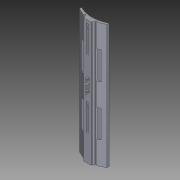
# Autodesk Inventor part: 3213_Bed Holder
Saved by Autodesk Inventor 2020 (Build 240168000, 168)
## iProperties
Created: 2019-06-26
Part Number: 3213_Bed Holder
Material: Acetal Resin, White
Document SubType Name: Sheet Metal
Designer: MPI
Density: 1.425 g/cm^3
Sheet Metal Rule: Default_mm
Appearance: Smooth - White
Mass: 236.302 g
Surface Area: 644.505 cm^2
Volume: 165.826 cm^3
Author: MPI
Autodesk Inventor part; units mm, degrees
sketch "Sketch1" plane through (0, 0, 0) normal (0, 0, 1) x (1, 0, 0)
  line L0 (0, 0) -> (-20.6965, 9.6509) construction
  line L1 (0, 0) -> (0, -60.6509) construction
  line L2 (0, 0) -> (-23.2307, -49.8183) construction
  line L3 (0, 0) -> (21.0241, 9.8037) construction
  line L4 (0, 0) -> (21.5225, -46.1553) construction
  line L5 (0, 0) -> (0, 48) construction
  arc A0 (-36, -19.5) -> (36, -19.5) centre (0, 48) ccw
  line L6 (-36, -19.5) -> (-36, -25.1413)
  line L7 (36, -19.5) -> (36, -25.1413)
  line L8 (-10, -40.5) -> (10, -40.5)
  line L9 (-10, -40.5) -> (-10, -37.2653)
  line L10 (10, -40.5) -> (10, -37.2653)
  line L11 (-17.6908, -33.679) -> (-16.0004, -30.0538)
  line L12 (-16.0004, -30.0538) -> (-12.7377, -31.5752)
  line L13 (-12.7377, -31.5752) -> (-14.4281, -35.2004)
  line L14 (14.4281, -35.2004) -> (12.7377, -31.5752)
  line L15 (12.7377, -31.5752) -> (16.0004, -30.0538)
  line L16 (16.0004, -30.0538) -> (17.6908, -33.679)
  line L17 (10, -37.2653) -> (14.4281, -35.2004)
  line L18 (17.6908, -33.679) -> (36, -25.1413)
  line L19 (-10, -37.2653) -> (-14.4281, -35.2004)
  line L20 (-17.6908, -33.679) -> (-36, -25.1413)
  dimension "d0" = 25
  dimension "d1" = 90
  dimension "d2" = 90
  dimension "d3" = 25
  dimension "d4" = 48
  dimension "d5" = 153
  dimension "d11" = 72
  dimension "d12" = 36
  dimension "d13" = 20
  dimension "d14" = 10
  dimension "d17" = 88.5
  dimension "d18" = 3.6
  dimension "d19" = 1.8
  dimension "d20" = 4
  dimension "d21" = 1.8
  dimension "d22" = 1.8
  dimension "d23" = 4
  constraints: 42 end point, 9 perpendicular, 5 parallel, 5 vertical, 2 point on circle, 1 centre point, 1 coincident, 1 horizontal
  measures "d0" angle of L1 L2
  measures "d1" angle of L2 L0
  measures "d2" angle of L4 L3
  measures "d3" angle of L1 L4
  measures "d4" distance of L0.start L5.end
  measures "d5" diameter of A0
  measures "d11" distance between parallel lines of L7 L6
  measures "d12" distance between parallel lines of L1 L6
  measures "d13" distance of L8.start L8.end
  measures "d14" distance between parallel lines of L1 L9
  measures "d17" distance from line of L8 L5.end
  measures "d18" distance between parallel lines of L11 L13
  measures "d19" distance from line of L2 L12.end
  measures "d20" distance of L12.end L13.end
  measures "d21" distance from line of L4 L14.end
  measures "d22" distance from line of L4 L15.end
  measures "d23" distance of L14.start L14.end
extrude "Extrusion1" add sketch "Sketch1" along normal blind 325
ref_plane "Work Plane1" through (0, 0, 60) normal (0, 0, -1) x (-1, 0, 0)
sketch "Sketch2" plane through (0, 0, 60) normal (0, 0, -1) x (-1, 0, 0)
  line L0 (14.4281, -35.2004) -> (12.7377, -31.5752)
  line L1 (12.7377, -31.5752) -> (16.0004, -30.0538)
  line L2 (14.4281, -35.2004) -> (10, -37.2653) projected
  line L3 (16.0004, -30.0538) -> (25.4652, -30.0538)
  line L4 (25.4652, -30.0538) -> (14.4281, -35.2004)
  line L5 (12.7377, -31.5752) -> (14.4281, -35.2004) projected
  line L6 (16.0004, -30.0538) -> (12.7377, -31.5752) projected
  line L7 (36, -25.1413) -> (17.6908, -33.679) projected
  line L8 (10, -40.5) -> (-10, -40.5) projected
  line L9 (-14.4281, -35.2004) -> (-12.7377, -31.5752)
  line L10 (-12.7377, -31.5752) -> (-16.0004, -30.0538)
  line L11 (-16.0004, -30.0538) -> (-25.4652, -30.0538)
  line L12 (-25.4652, -30.0538) -> (-14.4281, -35.2004)
  line L13 (-14.4281, -35.2004) -> (-12.7377, -31.5752) projected
  line L14 (-12.7377, -31.5752) -> (-16.0004, -30.0538) projected
  line L15 (-10, -37.2653) -> (-14.4281, -35.2004) projected
  line L16 (-17.6908, -33.679) -> (-36, -25.1413) projected
  point P0 (0, 0)
  constraints: 16 end point, 9 collinear, 3 parallel, 1 horizontal
extrude "Extrusion2" cut sketch "Sketch2" against normal blind 72
ref_plane "Work Plane2" through (0, 0, 192) normal (0, 0, -1) x (-1, 0, 0)
sketch "Sketch3" plane through (0, 0, 192) normal (0, 0, -1) x (-1, 0, 0)
  line L0 (14.4281, -35.2004) -> (12.7377, -31.5752)
  line L1 (12.7377, -31.5752) -> (14.4281, -35.2004) projected
  line L2 (12.7377, -31.5752) -> (16.0004, -30.0538)
  line L3 (16.0004, -30.0538) -> (25.4652, -30.0538)
  line L4 (25.4652, -30.0538) -> (14.4281, -35.2004)
  line L5 (-14.4281, -35.2004) -> (-12.7377, -31.5752)
  line L6 (-12.7377, -31.5752) -> (-16.0004, -30.0538)
  line L7 (-16.0004, -30.0538) -> (-25.4652, -30.0538)
  line L8 (-25.4652, -30.0538) -> (-14.4281, -35.2004)
  line L9 (16.0004, -30.0538) -> (12.7377, -31.5752) projected
  line L10 (14.4281, -35.2004) -> (10, -37.2653) projected
  line L11 (-14.4281, -35.2004) -> (-12.7377, -31.5752) projected
  line L12 (-12.7377, -31.5752) -> (-16.0004, -30.0538) projected
  line L13 (-10, -37.2653) -> (-14.4281, -35.2004) projected
  line L14 (10, -40.5) -> (-10, -40.5) projected
  line L15 (36, -25.1413) -> (17.6908, -33.679) projected
  point P0 (0, 0)
  constraints: 16 end point, 11 collinear, 2 parallel, 1 perpendicular
extrude "Extrusion3" cut sketch "Sketch3" against normal blind 73
ref_plane "Work Plane3" through (0, -25.1413, 0) normal (-1, 0, 0) x (0, 0, 1)
sketch "Sketch5" plane through (0, -25.1413, 0) normal (-1, 0, 0) x (0, 0, 1)
  line L0 (0, -7.5587) -> (0, -3.3587)
  line L1 (68, -7.5587) -> (68, -15.3587)
  line L2 (68, -15.3587) -> (138.7768, -15.3587)
  line L3 (138.7768, -15.3587) -> (108, -5.3587)
  line L4 (108, -5.3587) -> (108, -3.3587)
  line L5 (0, -15.3587) -> (325, -15.3587) projected
  line L6 (246, -7.5587) -> (246, -15.3587)
  line L7 (246, -15.3587) -> (316.7768, -15.3587)
  line L8 (68, -7.5587) -> (0, -7.5587)
  line L9 (286, -3.3587) -> (286, -5.3587)
  line L10 (316.7768, -15.3587) -> (286, -5.3587)
  line L11 (0, -3.3587) -> (0, -0.3587)
  line L12 (0, -8.5377) -> (0, 0) projected
  line L13 (0, 5.6413) -> (325, 5.6413) projected
  line L14 (286, -0.3587) -> (286, -3.3587)
  line L15 (246, -7.5587) -> (148, -7.5587)
  line L16 (148, -7.5587) -> (148, -3.3587)
  line L17 (108, -0.3587) -> (108, -3.3587)
  line L18 (325, -3.3587) -> (0, -3.3587) projected
  line L19 (148, -3.3587) -> (148, -0.3587)
  line L20 (0, -3.3587) -> (108, -3.3587)
  line L21 (148, -3.3587) -> (286, -3.3587)
  line L22 (0, -0.3587) -> (108, -0.3587)
  line L23 (148, -0.3587) -> (286, -0.3587)
  point P0 (0, 25.1413)
  dimension "d51" = 4.2
  dimension "d52" = 0
  dimension "d53" = 68
  dimension "d54" = 2
  dimension "d56" = 40
  dimension "d59" = 246
  dimension "d64" = 18
  dimension "d65" = 2
  dimension "d68" = 3
  dimension "d69" = 40
  dimension "d84" = 178
  dimension "d94" = 18
  dimension "d96" = 40
  constraints: 40 end point, 11 perpendicular, 4 parallel, 3 collinear, 3 horizontal, 2 vertical, 1 point on line
  measures "d51" distance of L0.start L0.end
  measures "d52" distance from line of L0 point (0, 25.141)
  measures "d53" distance between parallel lines of L1 L0
  measures "d54" distance of L3.end L4.end
  measures "d56" distance between parallel lines of L4 L1
  measures "d59" distance between parallel lines of L6 L0
  measures "d64" angle of L5 L10
  measures "d65" distance of L9.end L9.start
  measures "d68" distance of L0.end L11.end
  measures "d69" distance between parallel lines of L6 L9
  measures "d84" distance between parallel lines of L4 L9
  measures "d94" angle of L2 L3
  measures "d96" distance between parallel lines of L4 L16
extrude "Extrusion4" cut sketch "Sketch5" along normal mid plane 6.5 contours L0 L18 L4 L3 L2 L1 L8 | L11 L22 L17 L18 | L18 L9 L10 L5 L6 L15 L16 | L19 L23 L14 L18
sketch "Sketch6" plane through (-10, -40.5, 0) normal (0, -1, 0) x (1, 0, 0)
  line L0 (-49, 178) -> (79, 178) construction
  line L1 (10, 0) -> (10, 369) construction
  arc A0 (11, 159) -> (11, 169) centre (11, 164) ccw
  arc A1 (16, 183) -> (16, 173) centre (16, 178) ccw
  line L2 (11, 159) -> (11, 169)
  line L3 (16, 173) -> (16, 183)
  line L4 (11, 187) -> (11, 197)
  arc A2 (11, 187) -> (11, 197) centre (11, 192) ccw
  point P0 (4, 178)
  dimension "d70" = 178
  dimension "d85" = 1
  dimension "d86" = 5
  dimension "d87" = 5
  dimension "d88" = 6
  dimension "d89" = 5
  dimension "d90" = 1
  dimension "d91" = 14
  dimension "d92" = 14
  constraints: 10 end point, 6 point on circle, 3 centre point, 3 midpoint, 1 horizontal, 1 point on line, 1 vertical
  measures "d70" distance from line of L0 L1.start
  measures "d85" distance between parallel lines of L1 L2
  measures "d86" radius of A0
  measures "d87" radius of A1
  measures "d88" distance between parallel lines of L1 L3
  measures "d89" radius of A2
  measures "d90" distance between parallel lines of L1 L4
  measures "d91" vertical distance of A2.centre A1.centre
  measures "d92" vertical distance of A1.centre A0.centre
extrude "Extrusion5" add sketch "Sketch6" along normal blind 7
equation "\"BendRadius\" = Thickness"
equation "\"BendReliefWidth\" = Thickness"
equation "\"BendReliefDepth\" = 0.5 * Thickness"
equation "\"CornerReliefSize\" = 4 * Thickness"
equation "\"MinimumRemnant\" = 2 * Thickness"
equation "\"TransitionRadius\" = BendRadius"
equation "\"JacobiRadiusSize\" = BendRadius"
equation "\"GapSize\" = Thickness"
equation "\"Thickness\" = 0.5"
body "Solid1"
